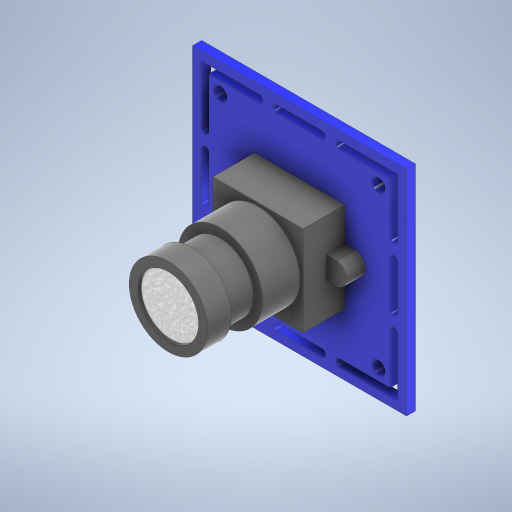
# Autodesk Inventor part: Camera2
Saved by Autodesk Inventor 2023 (Build 270158000, 158)
## iProperties
Created: 2023-05-07
Part Number: Camera2
Material: Generic
Document SubType Name: Modeling
Designer: karpova
Density: 1 g/cm^3
Appearance: Default
Author: karpova
Autodesk Inventor part; units mm, degrees
ref_plane "YZ Plane" through (0, 0, 0) normal (1, 0, 0) x (0, 1, 0)
ref_plane "XZ Plane" through (0, 0, 0) normal (0, 1, 0) x (-1, 0, 0)
ref_plane "XY Plane" through (0, 0, 0) normal (0, 0, 1) x (1, 0, 0)
sketch "Sketch1" plane through (0, 0, 0) normal (0, 0, 1) x (1, 0, 0)
  line L0 (0, 0) -> (38, 0)
  line L1 (38, 0) -> (38, 38)
  line L2 (38, 38) -> (0, 38)
  line L3 (0, 38) -> (0, 0)
  line L4 (35.1, 35.1) -> (2.9, 35.1)
  line L5 (0, 38) -> (38, 0) construction
  line L6 (38, 38) -> (0, 0) construction
  line L7 (19, 0) -> (19, 38) construction
  line L8 (0, 19) -> (38, 19) construction
  arc A0 (11.85, 1.6) -> (11.85, 2.9) centre (11.85, 2.25) ccw
  arc A1 (15.05, 2.9) -> (15.05, 1.6) centre (15.05, 2.25) ccw
  arc A2 (22.95, 1.6) -> (22.95, 2.9) centre (22.95, 2.25) ccw
  arc A3 (26.15, 2.9) -> (26.15, 1.6) centre (26.15, 2.25) ccw
  line L9 (2.9, 2.9) -> (11.85, 2.9)
  line L10 (11.85, 1.6) -> (1.6, 1.6)
  line L11 (36.4, 1.6) -> (26.15, 1.6)
  line L12 (22.95, 1.6) -> (15.05, 1.6)
  line L13 (15.05, 2.9) -> (22.95, 2.9)
  line L14 (26.15, 2.9) -> (35.1, 2.9)
  arc A4 (35.1, 26.15) -> (36.4, 26.15) centre (35.75, 26.15) ccw
  line L15 (35.1, 15.05) -> (35.1, 22.95)
  arc A5 (36.4, 22.95) -> (35.1, 22.95) centre (35.75, 22.95) ccw
  line L16 (36.4, 22.95) -> (36.4, 15.05)
  line L17 (36.4, 11.85) -> (36.4, 1.6)
  arc A6 (36.4, 11.85) -> (35.1, 11.85) centre (35.75, 11.85) ccw
  arc A7 (35.1, 15.05) -> (36.4, 15.05) centre (35.75, 15.05) ccw
  line L18 (35.1, 26.15) -> (35.1, 35.1)
  line L19 (36.4, 36.4) -> (36.4, 26.15)
  line L20 (35.1, 2.9) -> (35.1, 11.85)
  arc A8 (11.85, 35.1) -> (11.85, 36.4) centre (11.85, 35.75) ccw
  line L21 (22.95, 35.1) -> (15.05, 35.1)
  arc A9 (15.05, 36.4) -> (15.05, 35.1) centre (15.05, 35.75) ccw
  line L22 (15.05, 36.4) -> (22.95, 36.4)
  line L23 (26.15, 36.4) -> (36.4, 36.4)
  arc A10 (26.15, 36.4) -> (26.15, 35.1) centre (26.15, 35.75) ccw
  arc A11 (22.95, 35.1) -> (22.95, 36.4) centre (22.95, 35.75) ccw
  line L24 (11.85, 35.1) -> (2.9, 35.1)
  line L25 (1.6, 36.4) -> (11.85, 36.4)
  line L26 (35.1, 35.1) -> (26.15, 35.1)
  arc A12 (2.9, 11.85) -> (1.6, 11.85) centre (2.25, 11.85) ccw
  line L27 (2.9, 22.95) -> (2.9, 15.05)
  arc A13 (1.6, 15.05) -> (2.9, 15.05) centre (2.25, 15.05) ccw
  line L28 (1.6, 15.05) -> (1.6, 22.95)
  line L29 (1.6, 26.15) -> (1.6, 36.4)
  arc A14 (1.6, 26.15) -> (2.9, 26.15) centre (2.25, 26.15) ccw
  arc A15 (2.9, 22.95) -> (1.6, 22.95) centre (2.25, 22.95) ccw
  line L30 (2.9, 11.85) -> (2.9, 2.9)
  line L31 (1.6, 1.6) -> (1.6, 11.85)
  line L32 (2.9, 35.1) -> (2.9, 26.15)
  circle A16 centre (33.05, 4.95) radius 1.15
  line L33 (3.8, 34.2) -> (34.2, 34.2) construction
  line L34 (34.2, 34.2) -> (34.2, 3.8) construction
  line L35 (34.2, 3.8) -> (3.8, 3.8) construction
  line L36 (3.8, 3.8) -> (3.8, 34.2) construction
  circle A17 centre (4.95, 4.95) radius 1.15
  circle A18 centre (33.05, 33.05) radius 1.15
  circle A19 centre (4.95, 33.05) radius 1.15
  point P0 (23.6, 2.25)
  point P1 (14.4, 2.25)
  point P2 (25.5, 2.25)
  point P3 (12.5, 2.25)
  point P4 (19, 19)
  point P5 (35.75, 25.5)
  point P6 (35.75, 23.6)
  point P7 (35.75, 12.5)
  point P8 (35.75, 14.4)
  point P9 (12.5, 35.75)
  point P10 (14.4, 35.75)
  point P11 (25.5, 35.75)
  point P12 (23.6, 35.75)
  point P13 (2.25, 12.5)
  point P14 (2.25, 14.4)
  point P15 (2.25, 25.5)
  point P16 (2.25, 23.6)
  point P17 (2.9, 35.1)
  point P18 (26.15, 35.1)
  dimension "d0" = 38
  dimension "d1" = 38
  dimension "d4" = 9.2
  dimension "d5" = 13
  dimension "d8" = 360
  dimension "d10" = 2.3
  dimension "d11" = 0.9
  constraints: 74 end point, 36 point on circle, 28 tangent, 20 centre point, 7 parallel, 7 point on line, 5 midpoint, 3 equal radius, 2 horizontal, 2 perpendicular, 123 other
  measures "d0" distance of L0.end L1.end
  measures "d1" distance of L1.end L2.end
  measures "d4" distance of point (23.6, 2.25) point (14.4, 2.25)
  measures "d5" distance of point (25.5, 2.25) point (12.5, 2.25)
  measures "d10" diameter of A16
  measures "d11" distance between parallel lines of L14 L35
extrude "Extrusion1" add sketch "Sketch1" along normal blind 1.6
sketch "Sketch2" plane through (0, 0, 1.6) normal (0, 0, 1) x (1, 0, 0)
  line L0 (11, 27) -> (27, 27)
  line L1 (27, 27) -> (27, 11)
  line L2 (27, 11) -> (11, 11)
  line L3 (11, 11) -> (11, 27)
  line L4 (38, 38) -> (0, 38) construction
  line L5 (19, 38) -> (19, 0) construction
  line L6 (0, 0) -> (38, 0) construction
  line L7 (38, 0) -> (38, 38) construction
  line L8 (38, 19) -> (0, 19) construction
  line L9 (0, 38) -> (0, 0) construction
  dimension "d14" = 16
  dimension "d15" = 16
  constraints: 12 end point, 4 midpoint, 2 parallel, 1 horizontal, 1 perpendicular, 2 other
  measures "d14" distance of L0.start L0.end
  measures "d15" distance of L2.end L0.start
extrude "Extrusion2" add sketch "Sketch2" along normal blind 7.4
sketch "Sketch3" plane through (0, 0, 1.6) normal (0, 0, 1) x (1, 0, 0)
  line L0 (38, 38) -> (0, 38) construction
  line L1 (19, 38) -> (19, 0) construction
  line L2 (0, 0) -> (38, 0) construction
  line L3 (27, 11) -> (27, 27) projected
  line L4 (27, 21) -> (28.7765, 21)
  line L5 (28.7765, 17) -> (27, 17)
  line L6 (27, 17) -> (27, 21)
  arc A0 (28.7765, 17) -> (28.7765, 21) centre (28.6457, 19) ccw
  line L7 (0, 38) -> (0, 0) construction
  line L8 (0, 19) -> (38, 19) construction
  line L9 (38, 0) -> (38, 38) construction
  line L10 (11, 11) -> (11, 27)
  line L11 (11, 21) -> (9.2235, 21)
  line L12 (9.2235, 17) -> (11, 17)
  line L13 (11, 17) -> (11, 21)
  arc A1 (9.2235, 21) -> (9.2235, 17) centre (9.3543, 19) ccw
  line L14 (38, 19) -> (0, 19) construction
  point P0 (27.8883, 21)
  point P1 (10.1117, 21)
  point P2 (30.65, 19)
  point P3 (7.35, 19)
  dimension "d18" = 4
  dimension "d19" = 23.3
  constraints: 20 end point, 10 symmetric about line, 6 point on circle, 5 midpoint, 2 centre point, 2 point on line, 1 horizontal, 1 parallel, 2 other
  measures "d18" distance from line of point (27.888, 21) L5
  measures "d19" distance of point (30.65, 19) point (7.35, 19)
extrude "Extrusion3" add sketch "Sketch3" along normal blind 3.3
sketch "Sketch4" plane through (0, 0, 9) normal (0, 0, 1) x (1, 0, 0)
  line L0 (27, 27) -> (11, 27) construction
  line L1 (19, 27) -> (19, 11) construction
  line L2 (27, 11) -> (11, 11) construction
  line L3 (27, 11) -> (27, 27) construction
  line L4 (27, 19) -> (11, 19) construction
  line L5 (11, 27) -> (11, 11) construction
  circle A0 centre (19, 19) radius 7.5
  point P0 (0, 0)
  dimension "d22" = 15
  constraints: 5 midpoint, 4 end point, 1 centre point
  measures "d22" diameter of A0
extrude "Extrusion4" add sketch "Sketch4" along normal blind 6.7
sketch "Sketch5" plane through (19, 19, 15.7) normal (0, 0, 1) x (1, 0, 0)
  circle A0 centre (0, 0) radius 7.5 projected
  circle A1 centre (0, 0) radius 5.925
  point P0 (-19, -19)
  dimension "d25" = 11.85
  constraints: 1 centre point, 1 coincident
  measures "d25" diameter of A1
extrude "Extrusion5" add sketch "Sketch5" along normal blind 5 contours A1
sketch "Sketch6" plane through (19, 19, 20.7) normal (0, 0, 1) x (1, 0, 0)
  circle A0 centre (0, 0) radius 5.925 projected
  circle A1 centre (0, 0) radius 6.975
  point P0 (-19, -19)
  dimension "d28" = 13.95
  constraints: 1 centre point, 1 coincident
  measures "d28" diameter of A1
extrude "Extrusion6" add sketch "Sketch6" along normal blind 4.2 contours A0 | A1
sketch "Sketch7" plane through (19, 19, 24.9) normal (0, 0, 1) x (1, 0, 0)
  circle A0 centre (0, 0) radius 6.975 projected
  circle A1 centre (0, 0) radius 5.35
  point P0 (-19, -19)
  dimension "d31" = 10.7
  constraints: 1 centre point, 1 coincident
  measures "d31" diameter of A1
extrude "Extrusion7" cut sketch "Sketch7" against normal blind 0.5 contours A1
sketch "Sketch8" plane through (0, 0, 0) normal (0, 0, -1) x (-1, 0, 0)
  line L0 (-29.2, 8.2) -> (-19.15, 8.2)
  line L1 (-19.15, 8.2) -> (-19.15, 3.5)
  line L2 (-19.15, 3.5) -> (-29.2, 3.5)
  line L3 (-29.2, 3.5) -> (-29.2, 8.2)
  line L4 (-38, 0) -> (-38, 38) projected
  line L5 (0, 0) -> (-38, 0) projected
  dimension "d34" = 10.05
  dimension "d35" = 4.7
  dimension "d36" = 8.8
  dimension "d37" = 3.5
  constraints: 8 end point, 2 parallel, 1 horizontal, 1 perpendicular
  measures "d34" distance of L0.start L0.end
  measures "d35" distance of L0.end L1.end
  measures "d36" distance between parallel lines of L4 L3
  measures "d37" distance between parallel lines of L5 L2
extrude "Extrusion8" add sketch "Sketch8" along normal blind 6.2
sketch "Sketch9" plane through (0, 0, -6.2) normal (0, 0, -1) x (-1, 0, 0)
  line L0 (-29.2, 3.5) -> (-19.15, 3.5) projected
  line L1 (-19.15, 3.5) -> (-19.15, 8.2) projected
  line L2 (-19.15, 8.2) -> (-29.2, 8.2) projected
  line L3 (-29.2, 8.2) -> (-29.2, 3.5) projected
  line L4 (-28.7, 7.7) -> (-19.65, 7.7)
  line L5 (-19.65, 7.7) -> (-19.65, 4)
  line L6 (-19.65, 4) -> (-28.7, 4)
  line L7 (-28.7, 4) -> (-28.7, 7.7)
  point P0 (0, 0)
  dimension "d40" = 0.5
  constraints: 8 end point, 3 other
  measures "d40" distance between parallel lines of L2 L4
extrude "Extrusion9" cut sketch "Sketch9" against normal blind 4.8 contours L4 L5 L6 L7
sketch "Sketch10" plane through (0, 0, 0) normal (0, 0, -1) x (-1, 0, 0)
  line L0 (-34.35, 30.1061) -> (-3.65, 30.1061)
  line L1 (-3.65, 30.1061) -> (-3.65, 9.7)
  line L2 (-3.65, 9.7) -> (-34.35, 9.7)
  line L3 (-34.35, 9.7) -> (-34.35, 30.1061)
  line L4 (-2.9, 22.95) -> (-2.9, 15.05) projected
  line L5 (-35.1, 15.05) -> (-35.1, 22.95) projected
  line L6 (-35.1, 35.1) -> (-26.15, 35.1) projected
  line L7 (-27.85, 30.1061) -> (-16.55, 30.1061)
  line L8 (-16.55, 30.1061) -> (-16.55, 34.6)
  line L9 (-16.55, 34.6) -> (-27.85, 34.6)
  line L10 (-27.85, 34.6) -> (-27.85, 30.1061)
  line L11 (-18.15, 9.7) -> (-7.85, 9.7)
  line L12 (-7.85, 9.7) -> (-7.85, 3.65)
  line L13 (-7.85, 3.65) -> (-18.15, 3.65)
  line L14 (-18.15, 3.65) -> (-18.15, 9.7)
  line L15 (-19.15, 8.2) -> (-29.2, 8.2) projected
  line L16 (-19.15, 3.5) -> (-19.15, 8.2) projected
  line L17 (-15.05, 2.9) -> (-22.95, 2.9) projected
  line L18 (-22.95, 35.1) -> (-15.05, 35.1) projected
  line L19 (-38, 0) -> (-38, 38) projected
  point P0 (0, 0)
  dimension "d43" = 0.75
  dimension "d44" = 0.75
  dimension "d45" = 4.9939
  dimension "d46" = 1.5
  dimension "d47" = 1
  dimension "d48" = 0.75
  dimension "d49" = 10.3
  dimension "d50" = 0.5
  dimension "d51" = 10.15
  dimension "d52" = 11.3
  constraints: 24 end point, 6 parallel, 3 horizontal, 3 perpendicular, 2 point on line
  measures "d43" distance between parallel lines of L4 L1
  measures "d44" distance between parallel lines of L5 L3
  measures "d45" distance between parallel lines of L6 L0
  measures "d46" distance between parallel lines of L15 L2
  measures "d47" distance between parallel lines of L16 L14
  measures "d48" distance between parallel lines of L17 L13
  measures "d49" distance of L12.end L13.end
  measures "d50" distance between parallel lines of L18 L9
  measures "d51" distance between parallel lines of L19 L10
  measures "d52" distance of L8.end L9.end
extrude "Extrusion10" add sketch "Sketch10" along normal blind 2
body "Solid1"
